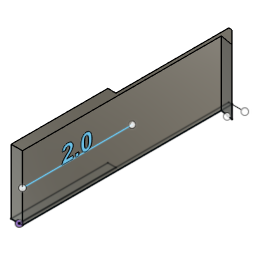
Door Locker V2 v20 (Autodesk Fusion 360 design; units mm, degrees)
Autodesk Fusion 360 part; units mm, degrees
sketch "Schizzo3" plane through (0, 0, 0) normal (0, 0, 1) x (1, 0, 0)
  line L0 (0, 0) -> (1, 0)
  line L1 (1, 0) -> (1, 65)
  line L2 (1, 65) -> (0, 65)
  line L3 (0, 65) -> (0, 0)
  line L4 (0, 0) -> (-2.5, 0)
  line L5 (-2.5, 0) -> (-2.5, 30)
  line L6 (-2.5, 30) -> (0, 30)
  line L7 (0, 30) -> (0, 0)
  line L8 (1, 65) -> (5, 61)
  line L9 (1, 65) -> (5, 65) construction
  line L10 (5, 61) -> (1, 61.7053)
  line L11 (5, 61) -> (3.5037, 61) construction
  dimension "d7" = 1
  dimension "d8" = 65
  dimension "d9" = 2.5
  dimension "d10" = 30
  dimension "d11" = 45
  dimension "d13" = 4
  dimension "d20" = 80
  constraint horizontal L0
  constraint vertical L1
  constraint horizontal L2
  constraint vertical L3
  constraint coincident L0.start L3.end
  constraint horizontal L4
  constraint vertical L5
  constraint horizontal L6
  constraint vertical L7
  constraint horizontal L9
  constraint horizontal L11
  constraint coincident L1 L10.end
  measures "d7" distance of L0.start L0.end
  measures "d8" distance of L0.start L2.end
  measures "d9" distance of L0.start L4.end
  measures "d10" distance of L0.start L6.end
  measures "d11" angle of L8 L9
  measures "d13" horizontal distance of L1.end L8.end
  measures "d20" angle of L1 L10
form "Forma1" [no effect]
extrude "Estrusione2" add sketch "Schizzo3" along normal blind 20
ref_plane "Piano di lavoro1" through (1, 30.8527, 10) normal (1, 0, 0) x (0, 1, 0)
sketch "Schizzo4" plane through (1, 0, 0) normal (1, 0, 0) x (0, 1, 0)
  line L0 (0, 10) -> (34, 10)
  dimension "d17" = 5
  text T0 "2.0" font "Arial" height 5 bold align centre spacing 1 along the path L0 letters at x, y, angle (12.145, 16.3233, 0) (16.0297, 16.3233, 0) (17.9703, 16.3233, 0)
  constraint horizontal L0
extrude "Estrusione3" cut sketch "Schizzo4" against normal blind 1 text T0
equation "d8 = 90 mm - 25 mm"
